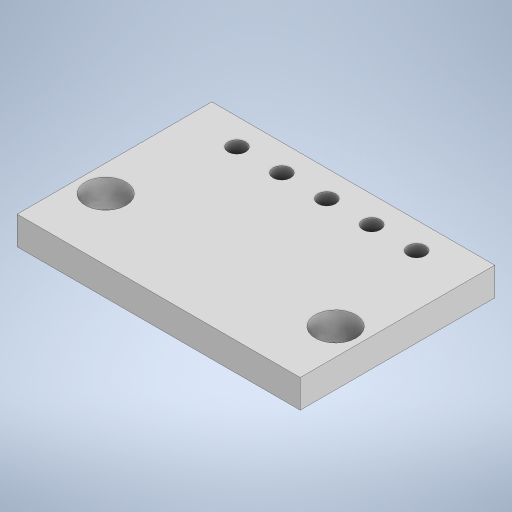
# Autodesk Inventor part: USB-C_BASE_plate
Saved by Autodesk Inventor 2024 (Build 280153000, 153)
## iProperties
Created: 2026-04-14
Part Number: USB-C_BASE_plate
Material: Generic
Document SubType Name: Modeling
Designer: Login
Density: 1 g/cm^3
Appearance: Default
Author: Login
Autodesk Inventor part; units mm, degrees
ref_plane "YZ Plane" through (0, 0, 0) normal (1, 0, 0) x (0, 1, 0)
ref_plane "XZ Plane" through (0, 0, 0) normal (0, 1, 0) x (-1, 0, 0)
ref_plane "XY Plane" through (0, 0, 0) normal (0, 0, 1) x (1, 0, 0)
sketch "Sketch1" plane through (0, 0, 0) normal (0, 1, 0) x (-1, 0, 0)
  line L0 (-8, 5.5) -> (8, 5.5)
  line L1 (8, 5.5) -> (8, -5.5)
  line L2 (8, -5.5) -> (-8, -5.5)
  line L3 (-8, -5.5) -> (-8, 5.5)
  line L4 (-8, 5.5) -> (8, -5.5) construction
  line L5 (8, 5.5) -> (-8, -5.5) construction
  point P0 (0, 0)
  dimension "d0" = 16
  dimension "d1" = 11
  constraints: 12 end point, 2 midpoint, 2 parallel, 1 horizontal, 1 perpendicular
  measures "d0" distance of L1.end L2.end
  measures "d1" distance of L0.end L1.end
extrude "Extrusion1" add sketch "Sketch1" along normal blind 1.6
sketch "Sketch2" plane through (0, 1.6, 0) normal (0, 1, 0) x (1, 0, 0)
  line L0 (8, -5.5) -> (8, 5.5) projected
  line L1 (-8, 5.5) -> (-8, -5.5) projected
  line L2 (8, 5.5) -> (-8, 5.5) projected
  point P0 (0, 0)
  point P1 (-6.5, -2)
  point P2 (6.5, -2)
  dimension "d4" = 1.5
  dimension "d5" = 1.5
  dimension "d6" = 7.5
  dimension "d7" = 7.5
  measures "d4" distance from line of L0 point (6.5, -2)
  measures "d5" distance from line of L1 point (-6.5, -2)
  measures "d6" distance from line of L2 point (6.5, -2)
  measures "d7" distance from line of L2 point (-6.5, -2)
hole "Hole1" at (-6.5, 1.6, 2) at (6.5, 1.6, 2) direction (0, -1, 0) diameter 2.3 end through all
sketch "Sketch3" plane through (0, 1.6, 0) normal (0, 1, 0) x (1, 0, 0)
  line L0 (-5.08, 4) -> (5.08, 4) construction
  line L1 (8, 5.5) -> (-8, 5.5) projected
  point P0 (0, 0)
  point P1 (0, 4)
  point P2 (-2.54, 4)
  point P3 (2.54, 4)
  point P4 (0, 4)
  dimension "d15" = 2.54
  dimension "d16" = 2.54
  dimension "d17" = 2.54
  dimension "d18" = 2.54
  dimension "d19" = 0
  dimension "d20" = 1.5
  constraints: 2 end point, 2 midpoint, 2 point on line, 1 horizontal
  measures "d15" distance of point (-2.54, 4) L0.start
  measures "d16" distance of point (0, 4) point (-2.54, 4)
  measures "d17" distance of point (2.54, 4) point (0, 4)
  measures "d18" distance of L0.end point (2.54, 4)
  measures "d19" horizontal distance of point (0, 0) point (0, 4)
  measures "d20" distance between parallel lines of L1 L0
hole "Hole2" at (0, 1.6, -4) at (-2.54, 1.6, -4) at (-5.08, 1.6, -4) at (2.54, 1.6, -4) at (5.08, 1.6, -4) direction (0, -1, 0) diameter 1 end through all
body "Solid1"
